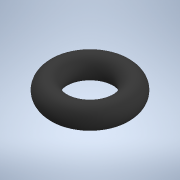
# Autodesk Inventor part: 103.018.01_Gummiring_Hubmagnet
Saved by Autodesk Inventor 2021 (Build 250183000, 183)
## iProperties
Created: 2021-12-02
Part Number: 103.018.01_Gummiring_Hubmagnet
Material: Gummi, Silikon
Document SubType Name: Modeling
Designer: Sebastian Seewald
Mass: 0.012337 g
Surface Area: 0.394784 cm^2
Volume: 0.0098696 cm^3
Density: 1.25 g/cm^3
Appearance: Gummi - Schwarz
Author: Sebastian Seewald
Autodesk Inventor part; units mm, degrees
ref_plane "YZ Plane" through (0, 0, 0) normal (1, 0, 0) x (0, 1, 0)
ref_plane "XZ Plane" through (0, 0, 0) normal (0, 1, 0) x (-1, 0, 0)
ref_plane "XY Plane" through (0, 0, 0) normal (0, 0, 1) x (1, 0, 0)
sketch "Skizze1" plane through (0, 0, 0) normal (0, 0, 1) x (1, 0, 0)
  circle A0 centre (2.8, 0) radius 1
  line L0 (0, -1.4) -> (0, 1.4) projected
  point P0 (0, 0)
  dimension "d0" = 2
  dimension "d1" = 2.8
  constraints: 1 centre point, 1 horizontal alignment
  measures "d0" diameter of A0
  measures "d1" distance of point (0, 0) A0.centre
revolve "Umdrehung1" add sketch "Skizze1" angle 360 about axis through (0, -10, 0) along (0, 1, 0)
